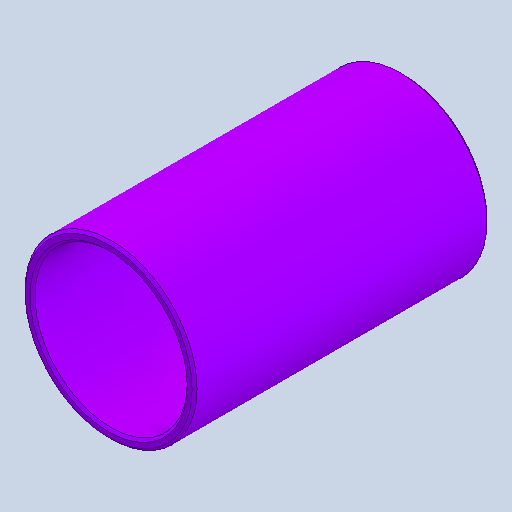
# Autodesk Inventor part: OutputBeltTensionerSleeve 5mm
Saved by Autodesk Inventor 2022.2 (Build 262287030, 287C)
## iProperties
Created: 2022-01-08
Part Number: OutputBeltTensionerSleeve 5mm
Material: Generic
Document SubType Name: Modeling
Designer: Jochen
Density: 1 g/cm^3
Appearance: Default
Author: Jochen
Autodesk Inventor part; units mm, degrees
ref_plane "YZ Plane" through (0, 0, 0) normal (1, 0, 0) x (0, 1, 0)
ref_plane "XZ Plane" through (0, 0, 0) normal (0, 1, 0) x (-1, 0, 0)
ref_plane "XY Plane" through (0, 0, 0) normal (0, 0, 1) x (1, 0, 0)
sketch "Sketch1" plane through (0, 0, 0) normal (0, 0, 1) x (1, 0, 0)
  line L0 (0, -2.45) -> (0, 2.45) construction
  line L1 (-2.45, 0) -> (2.45, 0) construction
  circle A0 centre (0, 0) radius 1.75
  circle A1 centre (0, 0) radius 1.55
  dimension "d0" = 3.5
  dimension "d1" = 0.2
  constraints: 2 centre point, 2 coincident
  measures "d0" diameter of A0
  measures "d1" radial gap between concentric circles of A0 A1
extrude "Extrusion1" add sketch "Sketch1" along normal blind 6
chamfer "Chamfer1" distance 0.05 angle 45 4 edges at (-1.75, 0, 6) (-1.55, 0, 6) (-1.75, 0, 0) (-1.55, 0, 0)
body "Solid1"
